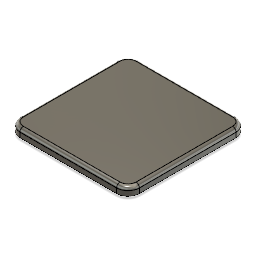
top_lid (Autodesk Fusion 360 design; units mm, degrees)
Autodesk Fusion 360 part; units mm, degrees
sketch "Sketch1" plane through (0, 0, 0) normal (0, 1, 0) x (1, 0, 0)
  line L0 (35.25, -35.25) -> (-35.25, -35.25)
  line L1 (-35.25, -35.25) -> (-35.25, 35.25)
  line L2 (-35.25, 35.25) -> (35.25, 35.25)
  line L3 (35.25, 35.25) -> (35.25, -35.25)
  line L4 (35.25, -35.25) -> (-35.25, 35.25) construction
  line L5 (-35.25, -35.25) -> (35.25, 35.25) construction
  dimension "d1" = 70.5
  dimension "d2" = 70.5
  constraint perpendicular L0 L1
  constraint parallel L0 L2
  constraint parallel L1 L3
  constraint horizontal L0
  constraint coincident L4 origin
  constraint coincident L5 origin
  measures "d1" distance of L1.end L2.end
  measures "d2" distance of L0.end L1.end
extrude "Extrude1" add sketch "Sketch1" along normal blind 5
sketch "Sketch2" plane through (0, 0, 0) normal (0, -1, 0) x (1, 0, 0)
  line L0 (-35.25, -35.25) -> (35.25, -35.25)
  line L1 (35.25, -35.25) -> (35.25, 35.25)
  line L2 (35.25, 35.25) -> (-35.25, 35.25)
  line L3 (-35.25, 35.25) -> (-35.25, -35.25)
  line L4 (32.95, -32.95) -> (32.95, 32.95)
  line L5 (32.95, 32.95) -> (-32.95, 32.95)
  line L6 (-32.95, 32.95) -> (-32.95, -32.95)
  line L7 (-32.95, -32.95) -> (32.95, -32.95)
  line L8 (32.95, 0) -> (30.95, 0)
  line L9 (0, -32.95) -> (0, -30.95)
  line L10 (-32.95, 0) -> (-30.95, 0)
  line L11 (0, 32.95) -> (0, 30.95)
  line L12 (-31.1, 31.1) -> (31.1, 31.1)
  line L13 (31.1, 31.1) -> (31.1, -31.1)
  line L14 (31.1, -31.1) -> (-31.1, -31.1)
  line L15 (-31.1, -31.1) -> (-31.1, 31.1)
  dimension "d5" = -2.3
  dimension "d6" = 2
  dimension "d7" = 2
  dimension "d8" = 2
  dimension "d9" = 2
  constraint midpoint L4 L8.start
  constraint perpendicular L4 L8
  constraint midpoint L7 L9.start
  constraint perpendicular L7 L9
  constraint midpoint L6 L10.start
  constraint perpendicular L6 L10
  constraint midpoint L5 L11.start
  constraint perpendicular L5 L11
  constraint horizontal L12
  constraint vertical L13
  constraint horizontal L14
  constraint vertical L15
  measures "d6" distance of L8.start L8.end
  measures "d7" distance of L9.start L9.end
  measures "d8" distance of L10.start L10.end
  measures "d9" distance of L11.start L11.end
extrude "Extrude2" add sketch "Sketch2" along normal blind 1.5 contours L4 L7 L8 L9 L13 L14 | L4 L5 L8 L11 L12 L13 | L6 L7 L9 L10 L14 L15 | L5 L6 L10 L11 L12 L15
fillet "Fillet1" radius 4.75 4 edges at (-32.95, -0.75, 32.95) (32.95, -0.75, 32.95) (32.95, -0.75, -32.95) (-32.95, -0.75, -32.95)
fillet "Fillet2" radius 3 4 edges at (31.1, -0.75, 31.1) (-31.1, -0.75, 31.1) (31.1, -0.75, -31.1) (-31.1, -0.75, -31.1)
fillet "Fillet3" radius 6.75 4 edges at (-35.25, 2.5, 35.25) (35.25, 2.5, 35.25) (35.25, 2.5, -35.25) (-35.25, 2.5, -35.25)
fillet "Fillet4" radius 2 8 edges at (-33.273, 5, -33.273) (-35.25, 5, 0) (-33.273, 5, 33.273) (0, 5, 35.25) (33.273, 5, 33.273) (35.25, 5, 0) (33.273, 5, -33.273) (0, 5, -35.25)
